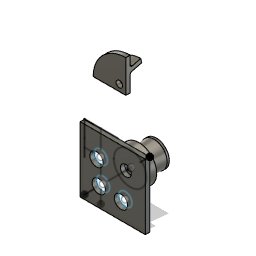
Coil Helpers v1 (Autodesk Fusion 360 design; units mm, degrees)
Autodesk Fusion 360 part; units mm, degrees
sketch "Sketch1" plane through (0, 0, 0) normal (0, 1, 0) x (1, 0, 0)
  line L0 (0, 0) -> (4.0226, 0)
  line L1 (4.747, 0.9441) -> (3.7059, 4.8296)
  line L2 (5, 0) -> (10, 0) construction
  arc A0 (4.0226, 0) -> (4.747, 0.9441) centre (4.0226, 0.75) ccw
  line L3 (7.7772, 0) -> (15, 0)
  line L4 (15, 0) -> (15, -2)
  line L5 (15, -2) -> (0, -2)
  line L6 (0, -2) -> (0, 0)
  line L7 (3.7059, 4.8296) -> (5.6378, 5.3473)
  line L8 (3.7059, 4.8296) -> (5.7059, 4.8296) construction
  line L9 (5.6378, 5.3473) -> (6.8081, 0.7531)
  arc A1 (6.8081, 0.7531) -> (7.7772, 0) centre (7.7772, 1) ccw
  dimension "d1" = 5
  dimension "d2" = 105
  dimension "d3" = 5
  dimension "d4" = 0.75
  dimension "d5" = 15
  dimension "d6" = 2
  dimension "d7" = 15
  dimension "d8" = 2
  dimension "d9" = 1
  constraint coincident L0.start L6.end
  constraint horizontal L0
  constraint horizontal L2
  constraint coincident L2.start L0
  constraint coincident L2.start L1
  constraint tangent L0 A0
  constraint tangent L1 A0
  constraint horizontal L3
  constraint vertical L4
  constraint horizontal L5
  constraint vertical L6
  constraint horizontal L8
  constraint coincident L0.start L3
  constraint tangent L9 A1
  constraint tangent L3 A1
  measures "d1" distance of L0.start L2.start
  measures "d2" angle of L1 L2
  measures "d3" distance of L2.start L1.end
  measures "d4" radius of A0
  measures "d5" distance of L0.start L3.end
  measures "d6" distance of L0.start L5.end
  measures "d7" angle of L7 L8
  measures "d8" distance of L1.end L7.end
  measures "d9" radius of A1
sketch "Sketch2" plane through (0, 0, 0) normal (0, 0, 1) x (1, 0, 0)
  line L0 (15, 0) -> (25, 0)
  circle A0 centre (25, 0) radius 10
  line L1 (25, 0) -> (25, -10)
  point P0 (15, 0)
  dimension "d10" = 10
  constraint coincident P0 L0.start
  constraint horizontal L0
  constraint coincident L0.end A0.centre
  constraint coincident P0 A0
  constraint coincident A0 L1.end
  constraint perpendicular L0 L1
  measures "d10" distance of P0 L0.end
revolve "Revolve1" add sketch "Sketch1" angle 90 about axis through (15, 0, 0) along (0, 0, -1) makes body 1
sketch "Sketch3" plane through (0, 0, 0) normal (0, 0, -1) x (-1, 0, 0)
  line L0 (-15, 0) -> (-7.7772, 0)
  arc A0 (-7.7772, 0) -> (-15, 7.2228) centre (-15, 0) ccw
  line L1 (-15, 7.2228) -> (-15, 0)
  line L2 (-15, 0) -> (-15, 3)
  line L3 (-15, 0) -> (-12, 0)
  line L4 (-15, 3) -> (-12, 0)
  line L5 (-12, 0) -> (-12, 8)
  line L6 (-15, 3.6114) -> (-7, 3.6114)
  line L7 (-15, 3) -> (-11, 3)
  circle A1 centre (-12, 3) radius 1.5
  dimension "d12" = 3
  dimension "d13" = 3
  dimension "d14" = 8
  dimension "d15" = 8
  dimension "d16" = 4
  dimension "d17" = 3
  constraint coincident L0.start A0.centre
  constraint perpendicular L0 L2
  constraint perpendicular L1 L3
  constraint perpendicular L0 L5
  constraint midpoint L1 L6.start
  constraint perpendicular L1 L6
  constraint perpendicular L2 L7
  constraint coincident L5 A1.centre
  constraint coincident L7 A1.centre
  measures "d12" distance of L0.start L2.end
  measures "d13" distance of L0.start L3.end
  measures "d14" distance of L3.end L5.end
  measures "d15" distance of L6.start L6.end
  measures "d16" distance of L2.end L7.end
  measures "d17" diameter of A1
hole "Hole1" at (12, 3, 0) direction (0, 0, 1) diameter 3 depth 5 tip angle 118 bodies 1
box "BoxPrimitive1" add length 30 width 30 height 2 placed x (0, -1, 0) y (1, 0, 0) z (0, 0, 1) at (-6, -21, 0) separate body makes body 2
sketch "Sketch7" plane through (0, 0, 2) normal (0, 0, 1) x (1, 0, 0)
  line L0 (-6, -51) -> (24, -51)
  line L1 (24, -51) -> (24, -21)
  line L2 (24, -21) -> (-6, -21)
  line L3 (-6, -21) -> (-6, -51)
  circle A0 through (20, -30, -2) (12.5, -25.6699, -2) (12.5, -34.3301, -2)
  dimension "d27" = 10
extrude "Extrude1" add sketch "Sketch7" against normal blind 2 contours A0 in plane through (0, 0, 0) normal (0, 0, 1) bodies 2
ref_plane "WorkPlane1" through (9, -36, 2) normal (0, 0, 1) x (1, 0, 0)
ref_plane "WorkPlane2" through (15, -30, -11) normal (0, 0, -1) x (-1, 0, 0)
cylinder "CylinderPrimitive1" add diameter 12 height 1 placed x (0, 1, 0) y (1, 0, 0) z (0, 0, -1) at (15, -30, -11) separate body makes body 3
loft "Loft1" add section 1 face at (13.3561, -30.7144, -11) section 2 face at (16.0062, -29.7035, -2) on bodies 2 3 bodies 3 2
shell "Shell1" thickness 2 removed faces 1 at (13.3561, -30.7144, -12) on bodies 3
sketch "Sketch10" plane through (0, 0, 0) normal (0, 0, -1) x (-1, 0, 0)
  circle A0 centre (-15, -30) radius 5
  line L0 (-24, -51) -> (6, -51)
  line L1 (6, -51) -> (6, -21)
  line L2 (6, -21) -> (-24, -21)
  line L3 (-24, -21) -> (-24, -51)
  line L4 (-24, -21) -> (-19.7927, -25.2073)
  line L5 (6, -51) -> (1.7927, -46.7927)
  line L6 (6, -51) -> (1.7927, -46.7927)
  line L7 (-4.6773, -40.3227) -> (-15.4794, -29.5206)
  line L8 (-19.7927, -25.2073) -> (-24, -21)
  circle A1 centre (-15, -30) radius 7.5
  line L9 (-9, -21) -> (6, -21)
  line L10 (6, -21) -> (6, -36)
  line L11 (6, -21) -> (6, -28.5)
  line L12 (6, -36) -> (6, -28.5)
  line L13 (6, -32.25) -> (1.55, -32.25)
  circle A2 centre (-1.5, -32.25) radius 3.05
  circle A3 centre (-12.75, -43.5) radius 3.05
  line L14 (-1.5, -21) -> (-1.5, -29.2)
  circle A4 centre (-2.5206, -42.4794) radius 3.05
  line L15 (-1.5, -35.3) -> (-1.5, -39.6052)
  line L16 (-1.5, -45.3536) -> (-1.5, -51)
  dimension "d40" = 15
  dimension "d43" = 6.1
  dimension "d44" = 6.1
  constraint coincident L0.end L1.start
  constraint coincident L2.end L3.start
  constraint parallel L4 L6
  constraint parallel L5 L6
  constraint collinear L6 L7
  constraint collinear L7 L8
  constraint concentric A0 A1
  constraint midpoint L2 L9.start
  constraint perpendicular L1 L9
  constraint midpoint L9 L14.start
  constraint coincident L0 L16.end
  constraint perpendicular L0 L14
  constraint midpoint L1 L10.end
  constraint perpendicular L2 L10
  constraint midpoint L10 L11.end
  constraint midpoint L12 L13.start
  constraint perpendicular L13 L14
  constraint symmetric L7 A2 A3
  constraint coincident A2 L14.end
  constraint collinear L14 L15
  constraint coincident A2 L15.start
  constraint coincident A2 L13.end
  constraint coincident A4 L15.end
  constraint coincident A4 L16.start
  constraint collinear L15 L16
  constraint coincident A4 L7.start
  measures "d40" diameter of A1
  measures "d43" diameter of A2
  measures "d44" diameter of A4
extrude "Extrude3" add sketch "Sketch10" along normal blind 4 draft 10 contours A1 bodies 3
cylinder "CylinderPrimitive2" cut diameter 5 height -7 placed x (0, 1, 0) y (1, 0, 0) z (0, 0, -1) at (15, -30, 0) bodies 3
move_face "OffsetFaces1" offset 3.1 1 faces at (15, -27, -0.7036) on bodies 3
extrude "Extrude4" cut sketch "Sketch10" against normal blind 3 contours A4 | A2 | A3 bodies 3
